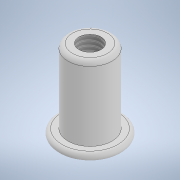
# Autodesk Inventor part: M3-RivetNut
Saved by Autodesk Inventor 2022.2 (Build 262287000, 287)
## iProperties
Created: 2022-03-31
Part Number: M3-RivetNut
Material: 一般
Document SubType Name: Modeling
Designer: Yuta Fujiyama
Density: 1 g/cm^3
Appearance: 既定
Author: Yuta Fujiyama
Autodesk Inventor part; units mm, degrees
ref_plane "YZ Plane" through (0, 0, 0) normal (1, 0, 0) x (0, 1, 0)
ref_plane "XZ Plane" through (0, 0, 0) normal (0, 1, 0) x (-1, 0, 0)
ref_plane "XY Plane" through (0, 0, 0) normal (0, 0, 1) x (1, 0, 0)
sketch "スケッチ1" plane through (0, 0, 0) normal (0, 1, 0) x (-1, 0, 0)
  circle A0 centre (0, 0) radius 3.5
  dimension "d0" = 7
  constraints: 1 centre point, 1 coincident
  measures "d0" diameter of A0
extrude "押し出し1" add sketch "スケッチ1" along normal blind 0.8
sketch "スケッチ2" plane through (0, 0.8, 0) normal (0, 1, 0) x (1, 0, 0)
  circle A0 centre (0, 0) radius 2.45
  dimension "d3" = 4.9
  constraints: 1 centre point, 1 coincident
  measures "d3" diameter of A0
extrude "押し出し2" add sketch "スケッチ2" along normal blind 8.2
fillet "フィレット1" radius 0.4 2 edges at (3.5, 0, 0) (3.5, 0.8, 0)
sketch "スケッチ3" plane through (0, 0, 0) normal (0, -1, 0) x (1, 0, 0)
  point P0 (0, 0)
  point P1 (0, 0)
  constraints: 1 coincident
hole "穴1" at (0, 0, 0) direction (0, 1, 0) diameter 2.459 end through all counterbore diameter 4.6 counterbore depth 5 thread size "M3x0.5" class "6H" standard "ISO Metric profile"
fillet "フィレット2" radius 0.2 2 edges at (0, 0, 2.3) (0, 5, 2.3)
fillet "フィレット2" radius 0.5 1 edges at (-2.45, 9, 0)
